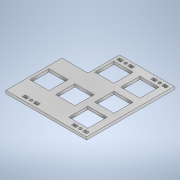
# Autodesk Inventor part: tc_base_plate
Saved by Autodesk Inventor 2020.1 (Build 241239000, 239)
## iProperties
Created: 2019-07-03
Part Number: tc_base_plate
Material: Acier inoxydable
Document SubType Name: Modeling
Designer: Thibault
Density: 8 g/cm^3
Appearance: Aluminium - Poli
Mass: 33.3223 g
Surface Area: 56.2435 cm^2
Volume: 4.16528 cm^3
tc_base_width: 59,100 mm
tc_base_back_width: 40,050 mm
tc_base_support_dist: 56,100 mm
Author: Thibault
Autodesk Inventor part; units mm, degrees
ref_plane "YZ Plane" through (0, 0, 0) normal (1, 0, 0) x (0, 1, 0)
ref_plane "XZ Plane" through (0, 0, 0) normal (0, 1, 0) x (-1, 0, 0)
ref_plane "XY Plane" through (0, 0, 0) normal (0, 0, 1) x (1, 0, 0)
sketch "screw_anchor" plane through (0, 0, 0) normal (0, 0, 1) x (1, 0, 0)
  point P0 (61.1245, 15.5217)
  dimension "d155" = 14
  dimension "d156" = 19.05
  dimension "d157" = 19.05
  dimension "d158" = 19.05
  dimension "d159" = 28.575
  dimension "d160" = 19.05
  dimension "d161" = 2
  dimension "d162" = 2
  dimension "d163" = 2
  dimension "d164" = 2
  dimension "d165" = 2
  dimension "d166" = 1
  dimension "d167" = 5
  dimension "d168" = 5
  dimension "d169" = 4
  dimension "tc_base_support_dist" = 56.1
sketch "anchor" plane through (0, 0, 0) normal (0, 0, 1) x (1, 0, 0)
  circle A0 centre (94.2814, 48.5827) radius 0.85
  line L0 (91.2814, 49.5827) -> (87.2814, 49.5827)
  line L1 (87.2814, 49.5827) -> (87.2814, 47.5827)
  line L2 (87.2814, 47.5827) -> (91.2814, 47.5827)
  line L3 (91.2814, 47.5827) -> (91.2814, 49.5827)
  line L4 (101.2814, 49.5827) -> (97.2814, 49.5827)
  line L5 (97.2814, 49.5827) -> (97.2814, 47.5827)
  line L6 (97.2814, 47.5827) -> (101.2814, 47.5827)
  line L7 (101.2814, 47.5827) -> (101.2814, 49.5827)
  line L8 (91.2814, 49.5827) -> (97.2814, 47.5827) construction
  line L9 (97.2814, 49.5827) -> (91.2814, 47.5827) construction
  line L10 (87.2814, 51.1827) -> (101.2814, 51.1827)
  point P0 (103.5798, 50.1132)
  point P1 (94.2814, 48.5827)
  dimension "tc_base_support_dist" = 56.1
  dimension "d226" = 1.7
  dimension "d230" = 4
  dimension "d231" = 2
  dimension "d237" = 4
  dimension "d245" = 1.6
  dimension "d247" = 6
  measures "d226" diameter of A0
  measures "d230" distance of L2.end L1.end
  measures "d231" distance of L1.end L0.end
  measures "d237" distance of L6.end L5.end
  measures "d245" distance between parallel lines of L0 L10
  measures "d247" distance between parallel lines of L5 L3
sketch "Anchor (screw side)" plane through (0, 0, 0) normal (0, 0, 1) x (1, 0, 0)
  circle A0 centre (93.7814, 50.2592) radius 1
  line L0 (91.2814, 51.2592) -> (88.2814, 51.2592)
  line L1 (88.2814, 51.2592) -> (88.2814, 49.2592)
  line L2 (88.2814, 49.2592) -> (91.2814, 49.2592)
  line L3 (91.2814, 49.2592) -> (91.2814, 51.2592)
  line L4 (99.2814, 51.2592) -> (96.2814, 51.2592)
  line L5 (96.2814, 51.2592) -> (96.2814, 49.2592)
  line L6 (96.2814, 49.2592) -> (99.2814, 49.2592)
  line L7 (99.2814, 49.2592) -> (99.2814, 51.2592)
  line L8 (91.2814, 51.2592) -> (96.2814, 49.2592) construction
  line L9 (96.2814, 51.2592) -> (91.2814, 49.2592) construction
  line L10 (86.2814, 53.2592) -> (101.2814, 53.2592) construction
  line L11 (101.2814, 53.2592) -> (101.2814, 47.2592) construction
  line L12 (101.2814, 47.2592) -> (86.2814, 47.2592) construction
  line L13 (86.2814, 47.2592) -> (86.2814, 53.2592) construction
  point P0 (103.5798, 50.1132)
  dimension "d27" = 2
  dimension "d28" = 3
  dimension "d29" = 2
  dimension "d30" = 3
  dimension "d32" = 5
  dimension "d34" = 2
  dimension "d35" = 2
  dimension "d36" = 2
  dimension "d37" = 2
  measures "d27" diameter of A0
  measures "d28" distance of L2.end L1.end
  measures "d29" distance of L1.end L0.end
  measures "d30" distance of L6.end L5.end
  measures "d32" distance between parallel lines of L5 L3
  measures "d34" distance between parallel lines of L0 L10
  measures "d35" distance between parallel lines of L12 L2
  measures "d36" distance between parallel lines of L11 L7
  measures "d37" distance between parallel lines of L13 L1
sketch "Anchor (nut side)" plane through (0, 0, 0) normal (0, 0, 1) x (1, 0, 0)
  line L0 (10, 0) -> (8.5, 0)
  line L1 (8.5, 0) -> (8.5, -2)
  line L2 (8.5, -2) -> (9.3, -2)
  line L3 (9.3, -2) -> (9.3, -4)
  line L4 (5.7, -4) -> (5.7, -2)
  line L5 (5.7, -2) -> (6.5, -2)
  line L6 (6.5, -2) -> (6.5, 0)
  line L7 (6.5, 0) -> (5, 0)
  line L8 (2, 0) -> (2, 2)
  line L9 (2, 0) -> (3, 0) construction
  line L10 (2, 2) -> (5, 2)
  line L11 (5, 2) -> (5, 0)
  line L12 (5, 2) -> (7, 2) construction
  line L13 (10, 0) -> (10, 2)
  line L14 (10, 2) -> (13, 2)
  line L15 (13, 2) -> (13, 0)
  line L16 (0, 0) -> (2, 0)
  line L17 (13, 0) -> (15, 0)
  line L18 (5.7, -4) -> (6.5, -4)
  line L19 (9.3, -4) -> (8.5, -4)
  line L20 (6.5, -4) -> (6.5, -6.25)
  line L21 (8.5, -4) -> (8.5, -6.25)
  line L22 (6.75, -6.5) -> (7.5, -6.5)
  arc A0 (6.5, -6.25) -> (6.75, -6.5) centre (6.75, -6.25) ccw
  arc A1 (8.25, -6.5) -> (8.5, -6.25) centre (8.25, -6.25) ccw
  line L23 (7.5, -7.2938) -> (7.5, -4.9797)
  line L24 (7.5, -6.5) -> (8.25, -6.5)
  point P0 (9.1321, -0.6227)
  point P1 (6.5, -6.5)
  point P2 (8.5, -6.5)
  dimension "d3" = 2
  dimension "d7" = 5
  dimension "d10" = 1.5
  dimension "d11" = 2
  dimension "d12" = 0.8
  dimension "d13" = 2
  dimension "d14" = 0.8
  dimension "d15" = 2
  dimension "d18" = 2
  dimension "d19" = 0.8
  dimension "d20" = 0.8
  dimension "d21" = 2.5
  dimension "d22" = 2.5
  dimension "d23" = 2
  dimension "d38" = 2
  dimension "d39" = 0.25
  dimension "d118" = 2
  dimension "d120" = 3
  measures "d3" distance of L16.start L8.start
  measures "d7" distance of L7.end L0.start
  measures "d10" distance of L0.start L0.end
  measures "d11" distance of L0.end L1.end
  measures "d12" distance of L1.end L2.end
  measures "d13" distance of L2.end L3.end
  measures "d14" distance of L4.end L5.end
  measures "d15" distance of L6.end L0.end
  measures "d18" distance of L15.end L17.end
  measures "d19" distance of L4.start L18.end
  measures "d20" distance of L3.end L19.end
  measures "d21" distance of L18.end point (6.5, -6.5)
  measures "d22" distance of L19.end point (8.5, -6.5)
  measures "d23" distance of L18.end L19.end
  measures "d38" distance between parallel lines of L16 L10
  measures "d39" radius of A0
  measures "d118" distance between parallel lines of L0 L14
  measures "d120" distance of L8.end L10.end
sketch "Screwless anchor (male)" plane through (0, 0, 0) normal (0, 0, 1) x (1, 0, 0)
  line L0 (1.6, 0) -> (1.6, 2)
  line L1 (1.6, 0) -> (2.6, 0) construction
  line L2 (1.6, 2) -> (4.6, 2)
  line L3 (4.6, 2) -> (4.6, 0)
  line L4 (9.6, 0) -> (9.6, 2)
  line L5 (9.6, 2) -> (12.6, 2)
  line L6 (12.6, 2) -> (12.6, 0)
  line L7 (0, 0) -> (1.6, 0)
  line L8 (12.6, 0) -> (14.2, 0)
  line L9 (4.6, 0) -> (9.6, 0)
  point P0 (9.1321, -0.6227)
  dimension "d81" = 1.6
  dimension "d83" = 5
  dimension "d92" = 1.6
  dimension "d100" = 2
  dimension "d119" = 3
  measures "d81" distance of L7.start L0.start
  measures "d83" distance of L3.end L4.start
  measures "d92" distance of L6.end L8.end
  measures "d100" distance between parallel lines of L7 L2
  measures "d119" distance of L0.end L2.end
sketch "Screwless anchor (female)" plane through (0, 0, 0) normal (0, 0, 1) x (1, 0, 0)
  line L0 (91.2814, 51.2592) -> (88.2814, 51.2592)
  line L1 (88.2814, 51.2592) -> (88.2814, 49.2592)
  line L2 (88.2814, 49.2592) -> (91.2814, 49.2592)
  line L3 (91.2814, 49.2592) -> (91.2814, 51.2592)
  line L4 (99.2814, 51.2592) -> (96.2814, 51.2592)
  line L5 (96.2814, 51.2592) -> (96.2814, 49.2592)
  line L6 (96.2814, 49.2592) -> (99.2814, 49.2592)
  line L7 (99.2814, 49.2592) -> (99.2814, 51.2592)
  line L8 (86.6814, 52.8592) -> (100.8814, 52.8592) construction
  line L9 (100.8814, 52.8592) -> (100.8814, 47.6592) construction
  line L10 (100.8814, 47.6592) -> (86.6814, 47.6592) construction
  line L11 (86.6814, 47.6592) -> (86.6814, 52.8592) construction
  point P0 (103.5798, 50.1132)
  dimension "d106" = 3
  dimension "d107" = 2
  dimension "d108_1" = 3
  dimension "d109_1" = 5
  dimension "d110_1" = 1.6
  dimension "d111_1" = 1.6
  dimension "d112" = 1.6
  dimension "d113" = 1.6
  measures "d106" distance of L2.end L1.end
  measures "d107" distance of L1.end L0.end
  measures "d108_1" distance of L6.end L5.end
  measures "d109_1" distance between parallel lines of L5 L3
  measures "d110_1" distance between parallel lines of L0 L8
  measures "d111_1" distance between parallel lines of L10 L2
  measures "d112" distance between parallel lines of L9 L7
  measures "d113" distance between parallel lines of L11 L1
sketch "Esquisse2" plane through (0, 0, 0) normal (0, 1, 0) x (-1, 0, 0)
  line L0 (17.4045, -3.6293) -> (3.4045, -3.6293)
  line L1 (3.4045, -3.6293) -> (3.4045, 10.3707)
  line L2 (3.4045, 10.3707) -> (17.4045, 10.3707)
  line L3 (17.4045, 10.3707) -> (17.4045, -3.6293)
  line L4 (17.4045, -41.7293) -> (3.4045, -41.7293)
  line L5 (3.4045, -41.7293) -> (3.4045, -27.7293)
  line L6 (3.4045, -27.7293) -> (17.4045, -27.7293)
  line L7 (17.4045, -27.7293) -> (17.4045, -41.7293)
  line L8 (17.4045, -22.6793) -> (3.4045, -22.6793)
  line L9 (3.4045, -22.6793) -> (3.4045, -8.6793)
  line L10 (3.4045, -8.6793) -> (17.4045, -8.6793)
  line L11 (17.4045, -8.6793) -> (17.4045, -22.6793)
  line L12 (36.4545, -41.7293) -> (22.4545, -41.7293)
  line L13 (22.4545, -41.7293) -> (22.4545, -27.7293)
  line L14 (22.4545, -27.7293) -> (36.4545, -27.7293)
  line L15 (36.4545, -27.7293) -> (36.4545, -41.7293)
  line L16 (36.4545, -13.1543) -> (22.4545, -13.1543)
  line L17 (22.4545, -13.1543) -> (22.4545, 0.8457)
  line L18 (22.4545, 0.8457) -> (36.4545, 0.8457)
  line L19 (36.4545, 0.8457) -> (36.4545, -13.1543)
  line L20 (55.5045, -13.1543) -> (41.5045, -13.1543)
  line L21 (41.5045, -13.1543) -> (41.5045, 0.8457)
  line L22 (41.5045, 0.8457) -> (55.5045, 0.8457)
  line L23 (55.5045, 0.8457) -> (55.5045, -13.1543)
  line L24 (57.5045, -24.6793) -> (38.4545, -24.6793)
  line L25 (38.4545, -24.6793) -> (38.4545, -47.7293)
  line L26 (38.4545, -47.7293) -> (-1.5955, -47.7293)
  line L27 (-1.5955, -47.7293) -> (-1.5955, 16.3707)
  line L28 (57.5045, -24.6793) -> (57.5045, 16.3707)
  line L29 (57.5045, 16.3707) -> (-1.5955, 16.3707)
  circle A0 centre (42.0045, 13.3707) radius 1
  line L30 (39.5045, 14.3707) -> (36.5045, 14.3707)
  line L31 (36.5045, 14.3707) -> (36.5045, 12.3707)
  line L32 (36.5045, 12.3707) -> (39.5045, 12.3707)
  line L33 (39.5045, 12.3707) -> (39.5045, 14.3707)
  line L34 (47.5045, 14.3707) -> (44.5045, 14.3707)
  line L35 (44.5045, 14.3707) -> (44.5045, 12.3707)
  line L36 (44.5045, 12.3707) -> (47.5045, 12.3707)
  line L37 (47.5045, 12.3707) -> (47.5045, 14.3707)
  line L38 (39.5045, 14.3707) -> (44.5045, 12.3707) construction
  line L39 (44.5045, 14.3707) -> (39.5045, 12.3707) construction
  line L40 (34.5045, 16.3707) -> (49.5045, 16.3707) construction
  line L41 (49.5045, 16.3707) -> (49.5045, 10.3707) construction
  line L42 (49.5045, 10.3707) -> (34.5045, 10.3707) construction
  line L43 (34.5045, 10.3707) -> (34.5045, 16.3707) construction
  circle A1 centre (5.9045, 13.3707) radius 1
  line L44 (3.4045, 14.3707) -> (0.4045, 14.3707)
  line L45 (0.4045, 14.3707) -> (0.4045, 12.3707)
  line L46 (0.4045, 12.3707) -> (3.4045, 12.3707)
  line L47 (3.4045, 12.3707) -> (3.4045, 14.3707)
  line L48 (11.4045, 14.3707) -> (8.4045, 14.3707)
  line L49 (8.4045, 14.3707) -> (8.4045, 12.3707)
  line L50 (8.4045, 12.3707) -> (11.4045, 12.3707)
  line L51 (11.4045, 12.3707) -> (11.4045, 14.3707)
  line L52 (3.4045, 14.3707) -> (8.4045, 12.3707) construction
  line L53 (8.4045, 14.3707) -> (3.4045, 12.3707) construction
  line L54 (-1.5955, 16.3707) -> (13.4045, 16.3707) construction
  line L55 (13.4045, 16.3707) -> (13.4045, 10.3707) construction
  line L56 (13.4045, 10.3707) -> (-1.5955, 10.3707) construction
  line L57 (-1.5955, 10.3707) -> (-1.5955, 16.3707) construction
  circle A2 centre (5.9045, -44.7293) radius 1
  line L58 (3.4045, -43.7293) -> (0.4045, -43.7293)
  line L59 (0.4045, -43.7293) -> (0.4045, -45.7293)
  line L60 (0.4045, -45.7293) -> (3.4045, -45.7293)
  line L61 (3.4045, -45.7293) -> (3.4045, -43.7293)
  line L62 (11.4045, -43.7293) -> (8.4045, -43.7293)
  line L63 (8.4045, -43.7293) -> (8.4045, -45.7293)
  line L64 (8.4045, -45.7293) -> (11.4045, -45.7293)
  line L65 (11.4045, -45.7293) -> (11.4045, -43.7293)
  line L66 (3.4045, -43.7293) -> (8.4045, -45.7293) construction
  line L67 (8.4045, -43.7293) -> (3.4045, -45.7293) construction
  line L68 (-1.5955, -41.7293) -> (13.4045, -41.7293) construction
  line L69 (13.4045, -41.7293) -> (13.4045, -47.7293) construction
  line L70 (13.4045, -47.7293) -> (-1.5955, -47.7293) construction
  line L71 (-1.5955, -47.7293) -> (-1.5955, -41.7293) construction
  circle A3 centre (30.9545, -44.7293) radius 1
  line L72 (28.4545, -43.7293) -> (25.4545, -43.7293)
  line L73 (25.4545, -43.7293) -> (25.4545, -45.7293)
  line L74 (25.4545, -45.7293) -> (28.4545, -45.7293)
  line L75 (28.4545, -45.7293) -> (28.4545, -43.7293)
  line L76 (36.4545, -43.7293) -> (33.4545, -43.7293)
  line L77 (33.4545, -43.7293) -> (33.4545, -45.7293)
  line L78 (33.4545, -45.7293) -> (36.4545, -45.7293)
  line L79 (36.4545, -45.7293) -> (36.4545, -43.7293)
  line L80 (28.4545, -43.7293) -> (33.4545, -45.7293) construction
  line L81 (33.4545, -43.7293) -> (28.4545, -45.7293) construction
  line L82 (23.4545, -41.7293) -> (38.4545, -41.7293) construction
  line L83 (38.4545, -41.7293) -> (38.4545, -47.7293) construction
  line L84 (38.4545, -47.7293) -> (23.4545, -47.7293) construction
  line L85 (23.4545, -47.7293) -> (23.4545, -41.7293) construction
  point P0 (39.3203, -53.3777)
  point P1 (31.7912, -47.7293)
  point P2 (1.2703, -53.3777)
  dimension "tc_base_support_dist" = 56.1
  dimension "d108" = 14
  dimension "d109" = 19.05
  dimension "d110" = 19.05
  dimension "d111" = 19.05
  dimension "d114" = 19.05
  dimension "d123" = 2
  dimension "d181" = 5
  dimension "d190" = 2
  dimension "d258" = 10
  dimension "d260" = 2
  dimension "d263" = 2
  dimension "d269" = 28.575
  dimension "d275" = 2
  constraints: 60 end point, 12 horizontal, 12 parallel, 11 equal length, 7 perpendicular, 6 vertical, 5 collinear, 3 point on line
  measures "d108" distance of L1.end L2.end
  measures "d109" distance of L8.end L4.end
  measures "d110" distance of L0.end L8.end
  measures "d111" distance of L4.start L12.start
  measures "d114" distance of L18.end L22.end
  measures "d123" distance between parallel lines of L8 L24
  measures "d181" distance between parallel lines of L27 L5
  measures "d190" distance between parallel lines of L28 L23
  measures "d269" distance between parallel lines of L16 L12
  measures "d275" distance between parallel lines of L25 L15
extrude "Base" add sketch "Esquisse2" along normal blind 2
ref_plane "Plan de construction4" through (-10.4045, 0, -41.7293) normal (-1, 0, 0) x (0, 0, 1)
ref_plane "Plan de construction5" through (-29.4545, 0, -27.7293) normal (1, 0, 0) x (0, 0, -1)
ref_plane "Plan de construction6" through (-48.5045, 0, -13.1543) normal (-1, 0, 0) x (0, 0, 1)
derived "shared_parameters.ipt"
